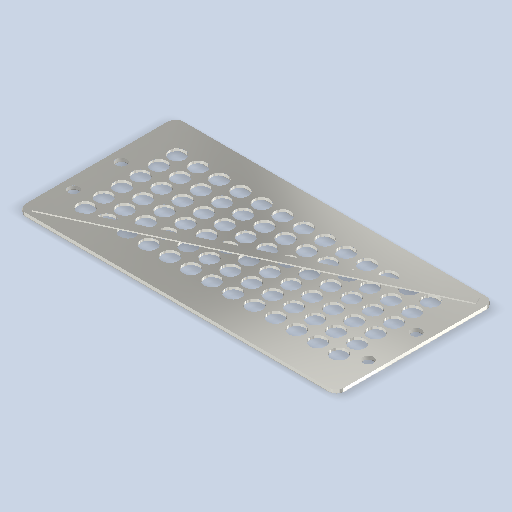
# Autodesk Inventor part: plate
Saved by Autodesk Inventor 2024 (Build 280153000, 153)
## iProperties
Created: 2024-04-23
Part Number: plate
Material: Eisen, Grau
Document SubType Name: Modeling
Designer: ffogue
Density: 7.15 g/cm^3
Appearance: Silber
Mass: 1548.48 g
Surface Area: 1353.02 cm^2
Volume: 216.571 cm^3
Author: ffogue
Autodesk Inventor part; units mm, degrees
ref_plane "YZ Plane" through (0, 0, 0) normal (1, 0, 0) x (0, 1, 0)
ref_plane "XZ Plane" through (0, 0, 0) normal (0, 1, 0) x (-1, 0, 0)
ref_plane "XY Plane" through (0, 0, 0) normal (0, 0, 1) x (1, 0, 0)
sketch "Skizze1" plane through (0, 0, 0) normal (0, 0, 1) x (1, 0, 0)
  line L0 (-200, -99) -> (200, -99)
  line L1 (200, -99) -> (200, 99)
  line L2 (200, 99) -> (-200, 99)
  line L3 (-200, 99) -> (-200, -99)
  line L4 (-200, -99) -> (200, 99) construction
  line L5 (200, -99) -> (-200, 99) construction
  point P0 (0, 0)
  dimension "d0" = 400
  dimension "d1" = 198
  constraints: 12 end point, 2 midpoint, 2 parallel, 1 horizontal, 1 perpendicular
  measures "d0" distance between parallel lines of L1 L3
  measures "d1" distance between parallel lines of L0 L2
extrude "Extrusion1" add sketch "Skizze1" along normal mid plane 4.5
sketch "Skizze2" plane through (0, 0, -2.25) normal (0, 0, -1) x (-1, 0, 0)
  line L0 (-170, -69) -> (170, -69)
  line L1 (170, -69) -> (170, 69)
  line L2 (170, 69) -> (-170, 69)
  line L3 (-170, 69) -> (-170, -69)
  line L4 (-170, -69) -> (170, 69) construction
  line L5 (170, -69) -> (-170, 69) construction
  line L6 (-200, 99) -> (-200, -99) projected
  line L7 (200, 99) -> (-200, 99) projected
  point P0 (0, 0)
  dimension "d4" = 30
  dimension "d5" = 30
  constraints: 12 end point, 2 midpoint, 2 parallel, 1 horizontal, 1 perpendicular
  measures "d4" distance between parallel lines of L3 L6
  measures "d5" distance between parallel lines of L7 L2
extrude "Extrusion2" cut sketch "Skizze2" against normal blind 1.5
sketch "Skizze3" plane through (0, 0, -0.75) normal (0, 0, -1) x (-1, 0, 0)
  circle A0 centre (-160, 59) radius 10
  line L0 (-170, 69) -> (170, 69) projected
  line L1 (-170, -69) -> (-170, 69) projected
  point P0 (0, 0)
  dimension "d8" = 20
  constraints: 2 tangent, 1 centre point
  measures "d8" diameter of A0
extrude "Extrusion3" cut sketch "Skizze3" against normal up to surface (3 mm away) contours A0
pattern_linear "Rechteckige Anordnung1" count 6 spacing 23 along (0, -1, 0) of "Extrusion3"
pattern_linear "Rechteckige Anordnung2" count 13 spacing 26.5 along (-1, 0, 0) of "Extrusion3", "Rechteckige Anordnung1"
fillet "Rundung1" radius 10 4 edges at (200, 99, 0) (-200, 99, 0) (-200, -99, 0) (200, -99, 0)
sketch "Skizze4" plane through (0, 0, -2.25) normal (0, 0, -1) x (-1, 0, 0)
  line L0 (-200, 89) -> (-200, -89) projected
  line L1 (200, -89) -> (200, 89) projected
  line L2 (-190, -99) -> (190, -99) projected
  point P0 (0, 0)
  point P1 (-185, -44)
  point P2 (-185, 16)
  point P3 (185, 16)
  point P4 (185, -44)
  dimension "d25" = 60
  dimension "d26" = 60
  dimension "d27" = 15
  dimension "d28" = 15
  dimension "d29" = 55
  constraints: 2 vertical alignment, 1 horizontal alignment
  measures "d25" distance of point (-185, -44) point (-185, 16)
  measures "d26" distance of point (185, -44) point (185, 16)
  measures "d27" distance from line of L0 point (-185, 16)
  measures "d28" distance from line of L1 point (185, 16)
  measures "d29" distance from line of L2 point (-185, -44)
hole "Bohrung1" at (185, -44, -2.25) at (185, 16, -2.25) at (-185, 16, -2.25) at (-185, -44, -2.25) direction (0, 0, 1) diameter 13.3762 depth 4.5 thread size "M15x1.5" class "6H" standard "ISO Metric profile"
sketch "Skizze6" plane through (0, 0, 2.25) normal (0, 0, 1) x (1, 0, 0)
  line L0 (190, 99) -> (-190, 99) projected
  arc A0 (-200, -89) -> (-190, -99) centre (-190, -89) ccw projected
  arc A1 (200, 89) -> (190, 99) centre (190, 89) ccw projected
  line L1 (190, 89) -> (-190, -89) construction
  line L2 (192.352, 83.9788) -> (-187.648, -94.0212)
  line L3 (-187.648, -94.0212) -> (-192.352, -83.9788)
  line L4 (-192.352, -83.9788) -> (187.648, 94.0212)
  line L5 (187.648, 94.0212) -> (192.352, 83.9788)
  point P0 (0, 0)
  point P1 (-190, -89)
  dimension "d33" = 10
  dimension "d34" = 10
  dimension "d35" = 419.6236
  constraints: 10 end point, 3 parallel, 2 midpoint, 1 coincident, 1 perpendicular, 1 other
  measures "d33" distance of L0.start point (190, 89)
  measures "d34" distance of A0.start point (-190, -89)
  measures "d35" distance of L1.start L1.end
extrude "Extrusion5" add sketch "Skizze6" along normal blind 1.5
equation "\"d5\" = d4"
